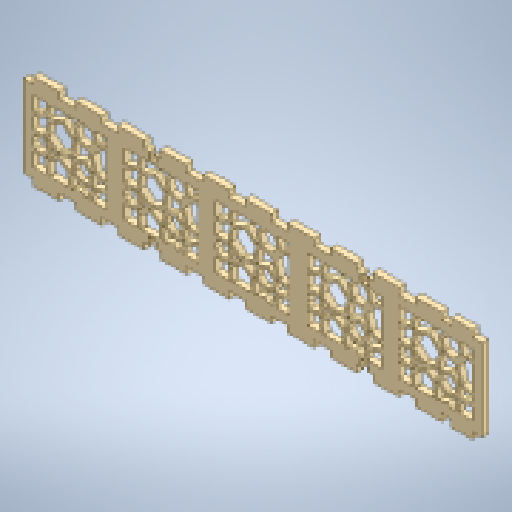
# Autodesk Inventor part: ширма
Saved by Autodesk Inventor 2023.1 (Build 271208000, 208)
## iProperties
Created: 2026-02-21
Part Number: ширма
Material: Типовые
Document SubType Name: Modeling
Designer: DELL
Density: 1 g/cm^3
Appearance: Пшеничный
Author: DELL
Autodesk Inventor part; units mm, degrees
ref_plane "YZ Plane" through (0, 0, 0) normal (1, 0, 0) x (0, 1, 0)
ref_plane "XZ Plane" through (0, 0, 0) normal (0, 1, 0) x (-1, 0, 0)
ref_plane "XY Plane" through (0, 0, 0) normal (0, 0, 1) x (1, 0, 0)
sketch "Эскиз1" plane through (0, 0, 0) normal (0, 0, 1) x (1, 0, 0)
  line L0 (-140.4, 25) -> (140.4, 25)
  line L1 (140.4, 25) -> (140.4, -25)
  line L2 (140.4, -25) -> (-140.4, -25)
  line L3 (-140.4, -25) -> (-140.4, 25)
  line L4 (-140.4, 25) -> (140.4, -25) construction
  line L5 (140.4, 25) -> (-140.4, -25) construction
  line L6 (-140.4, 0) -> (140.4, 0) construction
  line L7 (-140.4, 25) -> (-85.2, 25)
  line L8 (-85.2, 25) -> (-85.2, -25) construction
  line L9 (-85.2, -25) -> (-140.4, -25)
  line L10 (-140.4, -25) -> (-140.4, 25)
  line L11 (-89.2, -19) -> (-89.2, 19)
  line L12 (-89.2, 19) -> (-134.4, 19)
  line L13 (-134.4, 19) -> (-134.4, -19)
  line L14 (-134.4, -19) -> (-89.2, -19)
  line L15 (-125.4633, 11.2727) -> (-134.4, 8.1691)
  line L16 (-136.6237, 7.3969) -> (-145.5604, 15.1242) construction
  line L17 (-145.5604, 15.1242) -> (-143.3367, 26.7273) construction
  line L18 (-143.3367, 26.7273) -> (-132.1763, 30.6031) construction
  line L19 (-132.1763, 30.6031) -> (-123.2396, 22.8758) construction
  line L20 (-123.2396, 22.8758) -> (-123.9824, 19) construction
  line L21 (-127.2102, 12.7832) -> (-134.4, 10.2863)
  line L22 (-136.189, 9.665) -> (-143.3788, 15.8818) construction
  line L23 (-143.3788, 15.8818) -> (-141.5898, 25.2168) construction
  line L24 (-141.5898, 25.2168) -> (-132.611, 28.335) construction
  line L25 (-132.611, 28.335) -> (-125.4212, 22.1182) construction
  line L26 (-125.4212, 22.1182) -> (-126.0188, 19) construction
  line L27 (-107.9318, 7.9129) -> (-109.8716, -2.2089)
  line L28 (-109.8716, -2.2089) -> (-119.6072, -5.5899)
  line L29 (-119.6072, -5.5899) -> (-127.4031, 1.1509)
  line L30 (-127.4031, 1.1509) -> (-125.4633, 11.2727)
  line L31 (-125.4633, 11.2727) -> (-115.7276, 14.6537)
  line L32 (-115.7276, 14.6537) -> (-107.9318, 7.9129)
  line L33 (-116.1623, 12.3855) -> (-110.1134, 7.1552)
  line L34 (-110.1134, 7.1552) -> (-111.6185, -0.6984)
  line L35 (-111.6185, -0.6984) -> (-119.1726, -3.3218)
  line L36 (-119.1726, -3.3218) -> (-125.2215, 1.9085)
  line L37 (-125.2215, 1.9085) -> (-123.7163, 9.7622)
  line L38 (-123.7163, 9.7622) -> (-116.1623, 12.3855)
  line L39 (-102.8211, 0.2395) -> (-97.1755, -4.6421)
  line L40 (-97.1755, -4.6421) -> (-98.5803, -11.9722)
  line L41 (-98.5803, -11.9722) -> (-105.6307, -14.4207)
  line L42 (-105.6307, -14.4207) -> (-111.2764, -9.539)
  line L43 (-111.2764, -9.539) -> (-109.8716, -2.2089)
  line L44 (-109.8716, -2.2089) -> (-102.8211, 0.2395)
  line L45 (-103.2558, -2.0286) -> (-99.3571, -5.3997)
  line L46 (-99.3571, -5.3997) -> (-100.3272, -10.4617)
  line L47 (-100.3272, -10.4617) -> (-105.196, -12.1525)
  line L48 (-105.196, -12.1525) -> (-109.0948, -8.7814)
  line L49 (-109.0948, -8.7814) -> (-108.1247, -3.7194)
  line L50 (-108.1247, -3.7194) -> (-103.2558, -2.0286)
  line L51 (-98.5803, -11.9722) -> (-89.2, -8.7146)
  line L52 (-89.9827, -8.9864) -> (-83.0982, -14.9393) construction
  line L53 (-83.0982, -14.9393) -> (-84.8112, -23.8778) construction
  line L54 (-84.8112, -23.8778) -> (-93.4088, -26.8636) construction
  line L55 (-93.4088, -26.8636) -> (-102.5031, -19) construction
  line L56 (-100.2933, -20.9108) -> (-98.5803, -11.9722)
  line L57 (-90.4174, -11.2546) -> (-89.2, -12.3072)
  line L58 (-85.2798, -15.6969) -> (-86.5582, -22.3673) construction
  line L59 (-86.5582, -22.3673) -> (-92.9741, -24.5955) construction
  line L60 (-92.9741, -24.5955) -> (-99.4453, -19) construction
  line L61 (-98.1117, -20.1531) -> (-96.8333, -13.4827)
  line L62 (-96.8333, -13.4827) -> (-90.4174, -11.2546)
  line L63 (-110.531, -18.7283) -> (-110.9243, -19)
  line L64 (-118.1165, -23.9685) -> (-128.5977, -19) construction
  line L65 (-126.4473, -20.0194) -> (-127.1927, -10.8301)
  line L66 (-127.1927, -10.8301) -> (-119.6072, -5.5899)
  line L67 (-119.6072, -5.5899) -> (-111.2764, -9.539)
  line L68 (-111.2764, -9.539) -> (-110.531, -18.7283)
  line L69 (-118.3032, -21.6667) -> (-124.5472, -18.7068)
  line L70 (-124.5472, -18.7068) -> (-125.1059, -11.8193)
  line L71 (-125.1059, -11.8193) -> (-119.4205, -7.8918)
  line L72 (-119.4205, -7.8918) -> (-113.1765, -10.8517)
  line L73 (-113.1765, -10.8517) -> (-112.6178, -17.7391)
  line L74 (-112.6178, -17.7391) -> (-118.3032, -21.6667)
  line L75 (-104.7821, -16.8642) -> (-100.2933, -20.9108)
  line L76 (-100.2933, -20.9108) -> (-99.886, -19)
  line L77 (-101.5533, -26.8215) -> (-107.3022, -28.6856) construction
  line L78 (-107.3022, -28.6856) -> (-111.791, -24.6391) construction
  line L79 (-111.791, -24.6391) -> (-110.5889, -19)
  line L80 (-110.531, -18.7283) -> (-104.7821, -16.8642)
  line L81 (-105.2636, -19.1228) -> (-102.4901, -21.6231)
  line L82 (-102.4901, -21.6231) -> (-101.9309, -19)
  line L83 (-103.2686, -25.2752) -> (-106.8207, -26.427) construction
  line L84 (-106.8207, -26.427) -> (-109.5942, -23.9267) construction
  line L85 (-109.5942, -23.9267) -> (-108.544, -19) construction
  line L86 (-108.8157, -20.2746) -> (-105.2636, -19.1228)
  line L87 (-107.9318, 7.9129) -> (-110.126, 15.5167)
  line L88 (-110.126, 15.5167) -> (-106.7735, 19)
  line L89 (-104.6379, 21.2189) -> (-96.9557, 19.3171) construction
  line L90 (-96.9557, 19.3171) -> (-96.8642, 19)
  line L91 (-94.7615, 11.7133) -> (-100.2496, 6.0111)
  line L92 (-100.2496, 6.0111) -> (-107.9318, 7.9129)
  line L93 (-106.3303, 9.5768) -> (-107.8842, 14.9618)
  line L94 (-107.8842, 14.9618) -> (-103.9976, 19)
  line L95 (-103.9976, 19) -> (-98.5571, 17.6532)
  line L96 (-98.5571, 17.6532) -> (-97.0032, 12.2682)
  line L97 (-97.0032, 12.2682) -> (-100.8898, 8.23)
  line L98 (-100.8898, 8.23) -> (-106.3303, 9.5768)
  line L99 (-97.1755, -4.6421) -> (-100.2496, 6.0111)
  line L100 (-100.2496, 6.0111) -> (-92.5607, 14)
  line L101 (-92.5607, 14) -> (-89.2, 13.1681)
  line L102 (-81.7977, 11.3356) -> (-78.7236, 0.6824) construction
  line L103 (-78.7236, 0.6824) -> (-86.4125, -7.3065) construction
  line L104 (-86.4125, -7.3065) -> (-89.2, -6.6164) construction
  line L105 (-98.0078, 5.4562) -> (-91.9204, 11.7811)
  line L106 (-91.9204, 11.7811) -> (-89.2, 11.1077)
  line L107 (-83.3991, 9.6717) -> (-80.9653, 1.2373) construction
  line L108 (-80.9653, 1.2373) -> (-87.0528, -5.0876) construction
  line L109 (-87.0528, -5.0876) -> (-89.2, -4.556) construction
  line L110 (-95.574, -2.9782) -> (-98.0078, 5.4562)
  line L111 (-123.8393, -4.7789) -> (-127.1927, -10.8301)
  line L112 (-127.1927, -10.8301) -> (-134.1099, -10.9515)
  line L113 (-134.1099, -10.9515) -> (-134.4, -10.4689)
  line L114 (-137.6737, -5.0218) -> (-134.4, 0.8856) construction
  line L115 (-134.3203, 1.0294) -> (-127.4031, 1.1509)
  line L116 (-127.4031, 1.1509) -> (-123.8393, -4.7789)
  line L117 (-128.5225, -0.8691) -> (-126.1483, -4.8194)
  line L118 (-126.1483, -4.8194) -> (-128.3823, -8.8507)
  line L119 (-128.3823, -8.8507) -> (-132.9905, -8.9316)
  line L120 (-132.9905, -8.9316) -> (-134.4, -6.5863)
  line L121 (-135.3647, -4.9812) -> (-134.4, -3.2405) construction
  line L122 (-133.1306, -0.95) -> (-128.5225, -0.8691)
  line L123 (-134.4, 10.2863) -> (-136.189, 9.665) construction
  line L124 (-134.4, 8.1691) -> (-136.6237, 7.3969) construction
  line L125 (-126.0188, 19) -> (-127.2102, 12.7832)
  line L126 (-123.9824, 19) -> (-125.4633, 11.2727)
  line L127 (-106.7735, 19) -> (-104.6379, 21.2189) construction
  line L128 (-96.8642, 19) -> (-94.7615, 11.7133)
  line L129 (-89.2, 13.1681) -> (-81.7977, 11.3356) construction
  line L130 (-89.2, 11.1077) -> (-83.3991, 9.6717) construction
  line L131 (-89.2, -4.556) -> (-95.574, -2.9782)
  line L132 (-89.2, -6.6164) -> (-97.1755, -4.6421)
  line L133 (-89.2, -8.7146) -> (-89.9827, -8.9864) construction
  line L134 (-89.2, -12.3072) -> (-85.2798, -15.6969) construction
  line L135 (-99.4453, -19) -> (-98.1117, -20.1531)
  line L136 (-102.5031, -19) -> (-100.2933, -20.9108)
  line L137 (-99.886, -19) -> (-101.5533, -26.8215) construction
  line L138 (-101.9309, -19) -> (-103.2686, -25.2752) construction
  line L139 (-108.544, -19) -> (-108.8157, -20.2746)
  line L140 (-110.5889, -19) -> (-110.531, -18.7283)
  line L141 (-110.9243, -19) -> (-118.1165, -23.9685) construction
  line L142 (-128.5977, -19) -> (-126.4473, -20.0194)
  line L143 (-134.4, -10.4689) -> (-137.6737, -5.0218) construction
  line L144 (-134.4, -6.5863) -> (-135.3647, -4.9812) construction
  line L145 (-134.4, -3.2405) -> (-133.1306, -0.95)
  line L146 (-134.4, 0.8856) -> (-134.3203, 1.0294)
  line L147 (-72.5977, -19) -> (-70.4473, -20.0194)
  line L148 (-62.3032, -21.6667) -> (-68.5472, -18.7068)
  line L149 (-56.6178, -17.7391) -> (-62.3032, -21.6667)
  line L150 (-71.1927, -10.8301) -> (-63.6072, -5.5899)
  line L151 (-67.8393, -4.7789) -> (-71.1927, -10.8301)
  line L152 (-71.1927, -10.8301) -> (-78.1099, -10.9515)
  line L153 (-70.1483, -4.8194) -> (-72.3823, -8.8507)
  line L154 (-72.3823, -8.8507) -> (-76.9905, -8.9316)
  line L155 (-76.9905, -8.9316) -> (-78.4, -6.5863)
  line L156 (-78.1099, -10.9515) -> (-78.4, -10.4689)
  line L157 (-78.4, -3.2405) -> (-77.1306, -0.95)
  line L158 (-55.2764, -9.539) -> (-54.531, -18.7283)
  line L159 (-54.5889, -19) -> (-54.531, -18.7283)
  line L160 (-54.531, -18.7283) -> (-48.7821, -16.8642)
  line L161 (-52.544, -19) -> (-52.8157, -20.2746)
  line L162 (-52.8157, -20.2746) -> (-49.2636, -19.1228)
  line L163 (-78.3203, 1.0294) -> (-71.4031, 1.1509)
  line L164 (-78.4, 0.8856) -> (-78.3203, 1.0294)
  line L165 (-77.1306, -0.95) -> (-72.5225, -0.8691)
  line L166 (-72.5225, -0.8691) -> (-70.1483, -4.8194)
  line L167 (-63.1726, -3.3218) -> (-69.2215, 1.9085)
  line L168 (-63.6072, -5.5899) -> (-71.4031, 1.1509)
  line L169 (-71.4031, 1.1509) -> (-67.8393, -4.7789)
  line L170 (-53.8716, -2.2089) -> (-63.6072, -5.5899)
  line L171 (-55.6185, -0.6984) -> (-63.1726, -3.3218)
  line L172 (-49.6307, -14.4207) -> (-55.2764, -9.539)
  line L173 (-55.2764, -9.539) -> (-53.8716, -2.2089)
  line L174 (-63.6072, -5.5899) -> (-55.2764, -9.539)
  line L175 (-53.0948, -8.7814) -> (-52.1247, -3.7194)
  line L176 (-49.196, -12.1525) -> (-53.0948, -8.7814)
  line L177 (-63.4205, -7.8918) -> (-57.1765, -10.8517)
  line L178 (-69.2215, 1.9085) -> (-67.7163, 9.7622)
  line L179 (-71.4031, 1.1509) -> (-69.4633, 11.2727)
  line L180 (-67.7163, 9.7622) -> (-60.1623, 12.3855)
  line L181 (-69.4633, 11.2727) -> (-59.7276, 14.6537)
  line L182 (-69.4633, 11.2727) -> (-78.4, 8.1691)
  line L183 (-71.2102, 12.7832) -> (-78.4, 10.2863)
  line L184 (-42.5803, -11.9722) -> (-49.6307, -14.4207)
  line L185 (-44.3272, -10.4617) -> (-49.196, -12.1525)
  line L186 (-42.1117, -20.1531) -> (-40.8333, -13.4827)
  line L187 (-44.2933, -20.9108) -> (-42.5803, -11.9722)
  line L188 (-46.5031, -19) -> (-44.2933, -20.9108)
  line L189 (-44.2933, -20.9108) -> (-43.886, -19)
  line L190 (-46.4901, -21.6231) -> (-45.9309, -19)
  line L191 (-49.2636, -19.1228) -> (-46.4901, -21.6231)
  line L192 (-48.7821, -16.8642) -> (-44.2933, -20.9108)
  line L193 (-43.4453, -19) -> (-42.1117, -20.1531)
  line L194 (-78.4, 19) -> (-78.4, -19)
  line L195 (-41.1755, -4.6421) -> (-42.5803, -11.9722)
  line L196 (-43.3571, -5.3997) -> (-44.3272, -10.4617)
  line L197 (-42.5803, -11.9722) -> (-33.2, -8.7146)
  line L198 (-34.4174, -11.2546) -> (-33.2, -12.3072)
  line L199 (-40.8333, -13.4827) -> (-34.4174, -11.2546)
  line L200 (-51.9318, 7.9129) -> (-53.8716, -2.2089)
  line L201 (-59.7276, 14.6537) -> (-51.9318, 7.9129)
  line L202 (-60.1623, 12.3855) -> (-54.1134, 7.1552)
  line L203 (-54.1134, 7.1552) -> (-55.6185, -0.6984)
  line L204 (-50.3303, 9.5768) -> (-51.8842, 14.9618)
  line L205 (-51.9318, 7.9129) -> (-54.126, 15.5167)
  line L206 (-44.8898, 8.23) -> (-50.3303, 9.5768)
  line L207 (-44.2496, 6.0111) -> (-51.9318, 7.9129)
  line L208 (-41.0032, 12.2682) -> (-44.8898, 8.23)
  line L209 (-44.2496, 6.0111) -> (-36.5607, 14)
  line L210 (-53.8716, -2.2089) -> (-46.8211, 0.2395)
  line L211 (-52.1247, -3.7194) -> (-47.2558, -2.0286)
  line L212 (-47.2558, -2.0286) -> (-43.3571, -5.3997)
  line L213 (-46.8211, 0.2395) -> (-41.1755, -4.6421)
  line L214 (-42.0078, 5.4562) -> (-35.9204, 11.7811)
  line L215 (-40.8642, 19) -> (-38.7615, 11.7133)
  line L216 (-42.5571, 17.6532) -> (-41.0032, 12.2682)
  line L217 (-47.9976, 19) -> (-42.5571, 17.6532)
  line L218 (-40.9557, 19.3171) -> (-40.8642, 19)
  line L219 (-51.8842, 14.9618) -> (-47.9976, 19)
  line L220 (-54.126, 15.5167) -> (-50.7735, 19)
  line L221 (-38.7615, 11.7133) -> (-44.2496, 6.0111)
  line L222 (-33.2, -6.6164) -> (-41.1755, -4.6421)
  line L223 (-33.2, -4.556) -> (-39.574, -2.9782)
  line L224 (-41.1755, -4.6421) -> (-44.2496, 6.0111)
  line L225 (-39.574, -2.9782) -> (-42.0078, 5.4562)
  line L226 (-35.9204, 11.7811) -> (-33.2, 11.1077)
  line L227 (-36.5607, 14) -> (-33.2, 13.1681)
  line L228 (-68.5472, -18.7068) -> (-69.1059, -11.8193)
  line L229 (-54.531, -18.7283) -> (-54.9243, -19)
  line L230 (-69.1059, -11.8193) -> (-63.4205, -7.8918)
  line L231 (-57.1765, -10.8517) -> (-56.6178, -17.7391)
  line L232 (-78.4, -19) -> (-33.2, -19)
  line L233 (-33.2, -19) -> (-33.2, 19)
  line L234 (-33.2, 19) -> (-78.4, 19)
  line L235 (-70.4473, -20.0194) -> (-71.1927, -10.8301)
  line L236 (-67.9824, 19) -> (-69.4633, 11.2727)
  line L237 (-70.0188, 19) -> (-71.2102, 12.7832)
  line L238 (-16.5977, -19) -> (-14.4473, -20.0194)
  line L239 (-6.3032, -21.6667) -> (-12.5472, -18.7068)
  line L240 (-0.6178, -17.7391) -> (-6.3032, -21.6667)
  line L241 (-15.1927, -10.8301) -> (-7.6072, -5.5899)
  line L242 (-11.8393, -4.7789) -> (-15.1927, -10.8301)
  line L243 (-15.1927, -10.8301) -> (-22.1099, -10.9515)
  line L244 (-14.1483, -4.8194) -> (-16.3823, -8.8507)
  line L245 (-16.3823, -8.8507) -> (-20.9905, -8.9316)
  line L246 (-20.9905, -8.9316) -> (-22.4, -6.5863)
  line L247 (-22.1099, -10.9515) -> (-22.4, -10.4689)
  line L248 (-22.4, -3.2405) -> (-21.1306, -0.95)
  line L249 (0.7236, -9.539) -> (1.469, -18.7283)
  line L250 (1.4111, -19) -> (1.469, -18.7283)
  line L251 (1.469, -18.7283) -> (7.2179, -16.8642)
  line L252 (3.456, -19) -> (3.1843, -20.2746)
  line L253 (3.1843, -20.2746) -> (6.7364, -19.1228)
  line L254 (-22.3203, 1.0294) -> (-15.4031, 1.1509)
  line L255 (-22.4, 0.8856) -> (-22.3203, 1.0294)
  line L256 (-21.1306, -0.95) -> (-16.5225, -0.8691)
  line L257 (-16.5225, -0.8691) -> (-14.1483, -4.8194)
  line L258 (-7.1726, -3.3218) -> (-13.2215, 1.9085)
  line L259 (-7.6072, -5.5899) -> (-15.4031, 1.1509)
  line L260 (-15.4031, 1.1509) -> (-11.8393, -4.7789)
  line L261 (2.1284, -2.2089) -> (-7.6072, -5.5899)
  line L262 (0.3815, -0.6984) -> (-7.1726, -3.3218)
  line L263 (6.3693, -14.4207) -> (0.7236, -9.539)
  line L264 (0.7236, -9.539) -> (2.1284, -2.2089)
  line L265 (-7.6072, -5.5899) -> (0.7236, -9.539)
  line L266 (2.9052, -8.7814) -> (3.8753, -3.7194)
  line L267 (6.804, -12.1525) -> (2.9052, -8.7814)
  line L268 (-7.4205, -7.8918) -> (-1.1765, -10.8517)
  line L269 (-13.2215, 1.9085) -> (-11.7163, 9.7622)
  line L270 (-15.4031, 1.1509) -> (-13.4633, 11.2727)
  line L271 (-11.7163, 9.7622) -> (-4.1623, 12.3855)
  line L272 (-13.4633, 11.2727) -> (-3.7276, 14.6537)
  line L273 (-13.4633, 11.2727) -> (-22.4, 8.1691)
  line L274 (-15.2102, 12.7832) -> (-22.4, 10.2863)
  line L275 (13.4197, -11.9722) -> (6.3693, -14.4207)
  line L276 (11.6728, -10.4617) -> (6.804, -12.1525)
  line L277 (13.8883, -20.1531) -> (15.1667, -13.4827)
  line L278 (11.7067, -20.9108) -> (13.4197, -11.9722)
  line L279 (9.4969, -19) -> (11.7067, -20.9108)
  line L280 (11.7067, -20.9108) -> (12.114, -19)
  line L281 (9.5099, -21.6231) -> (10.0691, -19)
  line L282 (6.7364, -19.1228) -> (9.5099, -21.6231)
  line L283 (7.2179, -16.8642) -> (11.7067, -20.9108)
  line L284 (12.5547, -19) -> (13.8883, -20.1531)
  line L285 (-22.4, 19) -> (-22.4, -19)
  line L286 (14.8245, -4.6421) -> (13.4197, -11.9722)
  line L287 (12.6429, -5.3997) -> (11.6728, -10.4617)
  line L288 (13.4197, -11.9722) -> (22.8, -8.7146)
  line L289 (21.5826, -11.2546) -> (22.8, -12.3072)
  line L290 (15.1667, -13.4827) -> (21.5826, -11.2546)
  line L291 (4.0682, 7.9129) -> (2.1284, -2.2089)
  line L292 (-3.7276, 14.6537) -> (4.0682, 7.9129)
  line L293 (-4.1623, 12.3855) -> (1.8866, 7.1552)
  line L294 (1.8866, 7.1552) -> (0.3815, -0.6984)
  line L295 (5.6697, 9.5768) -> (4.1158, 14.9618)
  line L296 (4.0682, 7.9129) -> (1.874, 15.5167)
  line L297 (11.1102, 8.23) -> (5.6697, 9.5768)
  line L298 (11.7504, 6.0111) -> (4.0682, 7.9129)
  line L299 (14.9968, 12.2682) -> (11.1102, 8.23)
  line L300 (11.7504, 6.0111) -> (19.4393, 14)
  line L301 (2.1284, -2.2089) -> (9.1789, 0.2395)
  line L302 (3.8753, -3.7194) -> (8.7442, -2.0286)
  line L303 (8.7442, -2.0286) -> (12.6429, -5.3997)
  line L304 (9.1789, 0.2395) -> (14.8245, -4.6421)
  line L305 (13.9922, 5.4562) -> (20.0796, 11.7811)
  line L306 (15.1358, 19) -> (17.2385, 11.7133)
  line L307 (13.4429, 17.6532) -> (14.9968, 12.2682)
  line L308 (8.0024, 19) -> (13.4429, 17.6532)
  line L309 (15.0443, 19.3171) -> (15.1358, 19)
  line L310 (4.1158, 14.9618) -> (8.0024, 19)
  line L311 (1.874, 15.5167) -> (5.2265, 19)
  line L312 (17.2385, 11.7133) -> (11.7504, 6.0111)
  line L313 (22.8, -6.6164) -> (14.8245, -4.6421)
  line L314 (22.8, -4.556) -> (16.426, -2.9782)
  line L315 (14.8245, -4.6421) -> (11.7504, 6.0111)
  line L316 (16.426, -2.9782) -> (13.9922, 5.4562)
  line L317 (20.0796, 11.7811) -> (22.8, 11.1077)
  line L318 (19.4393, 14) -> (22.8, 13.1681)
  line L319 (-12.5472, -18.7068) -> (-13.1059, -11.8193)
  line L320 (1.469, -18.7283) -> (1.0757, -19)
  line L321 (-13.1059, -11.8193) -> (-7.4205, -7.8918)
  line L322 (-1.1765, -10.8517) -> (-0.6178, -17.7391)
  line L323 (-22.4, -19) -> (22.8, -19)
  line L324 (22.8, -19) -> (22.8, 19)
  line L325 (22.8, 19) -> (-22.4, 19)
  line L326 (-14.4473, -20.0194) -> (-15.1927, -10.8301)
  line L327 (-11.9824, 19) -> (-13.4633, 11.2727)
  line L328 (-14.0188, 19) -> (-15.2102, 12.7832)
  line L329 (39.4023, -19) -> (41.5527, -20.0194)
  line L330 (49.6968, -21.6667) -> (43.4528, -18.7068)
  line L331 (55.3822, -17.7391) -> (49.6968, -21.6667)
  line L332 (40.8073, -10.8301) -> (48.3928, -5.5899)
  line L333 (44.1607, -4.7789) -> (40.8073, -10.8301)
  line L334 (40.8073, -10.8301) -> (33.8901, -10.9515)
  line L335 (41.8517, -4.8194) -> (39.6177, -8.8507)
  line L336 (39.6177, -8.8507) -> (35.0095, -8.9316)
  line L337 (35.0095, -8.9316) -> (33.6, -6.5863)
  line L338 (33.8901, -10.9515) -> (33.6, -10.4689)
  line L339 (33.6, -3.2405) -> (34.8694, -0.95)
  line L340 (56.7236, -9.539) -> (57.469, -18.7283)
  line L341 (57.4111, -19) -> (57.469, -18.7283)
  line L342 (57.469, -18.7283) -> (63.2179, -16.8642)
  line L343 (59.456, -19) -> (59.1843, -20.2746)
  line L344 (59.1843, -20.2746) -> (62.7364, -19.1228)
  line L345 (33.6797, 1.0294) -> (40.5969, 1.1509)
  line L346 (33.6, 0.8856) -> (33.6797, 1.0294)
  line L347 (34.8694, -0.95) -> (39.4775, -0.8691)
  line L348 (39.4775, -0.8691) -> (41.8517, -4.8194)
  line L349 (48.8274, -3.3218) -> (42.7785, 1.9085)
  line L350 (48.3928, -5.5899) -> (40.5969, 1.1509)
  line L351 (40.5969, 1.1509) -> (44.1607, -4.7789)
  line L352 (58.1284, -2.2089) -> (48.3928, -5.5899)
  line L353 (56.3815, -0.6984) -> (48.8274, -3.3218)
  line L354 (62.3693, -14.4207) -> (56.7236, -9.539)
  line L355 (56.7236, -9.539) -> (58.1284, -2.2089)
  line L356 (48.3928, -5.5899) -> (56.7236, -9.539)
  line L357 (58.9052, -8.7814) -> (59.8753, -3.7194)
  line L358 (62.804, -12.1525) -> (58.9052, -8.7814)
  line L359 (48.5795, -7.8918) -> (54.8235, -10.8517)
  line L360 (42.7785, 1.9085) -> (44.2837, 9.7622)
  line L361 (40.5969, 1.1509) -> (42.5367, 11.2727)
  line L362 (44.2837, 9.7622) -> (51.8377, 12.3855)
  line L363 (42.5367, 11.2727) -> (52.2724, 14.6537)
  line L364 (42.5367, 11.2727) -> (33.6, 8.1691)
  line L365 (40.7898, 12.7832) -> (33.6, 10.2863)
  line L366 (69.4197, -11.9722) -> (62.3693, -14.4207)
  line L367 (67.6728, -10.4617) -> (62.804, -12.1525)
  line L368 (69.8883, -20.1531) -> (71.1667, -13.4827)
  line L369 (67.7067, -20.9108) -> (69.4197, -11.9722)
  line L370 (65.4969, -19) -> (67.7067, -20.9108)
  line L371 (67.7067, -20.9108) -> (68.114, -19)
  line L372 (65.5099, -21.6231) -> (66.0691, -19)
  line L373 (62.7364, -19.1228) -> (65.5099, -21.6231)
  line L374 (63.2179, -16.8642) -> (67.7067, -20.9108)
  line L375 (68.5547, -19) -> (69.8883, -20.1531)
  line L376 (33.6, 19) -> (33.6, -19)
  line L377 (70.8245, -4.6421) -> (69.4197, -11.9722)
  line L378 (68.6429, -5.3997) -> (67.6728, -10.4617)
  line L379 (69.4197, -11.9722) -> (78.8, -8.7146)
  line L380 (77.5826, -11.2546) -> (78.8, -12.3072)
  line L381 (71.1667, -13.4827) -> (77.5826, -11.2546)
  line L382 (60.0682, 7.9129) -> (58.1284, -2.2089)
  line L383 (52.2724, 14.6537) -> (60.0682, 7.9129)
  line L384 (51.8377, 12.3855) -> (57.8866, 7.1552)
  line L385 (57.8866, 7.1552) -> (56.3815, -0.6984)
  line L386 (61.6697, 9.5768) -> (60.1158, 14.9618)
  line L387 (60.0682, 7.9129) -> (57.874, 15.5167)
  line L388 (67.1102, 8.23) -> (61.6697, 9.5768)
  line L389 (67.7504, 6.0111) -> (60.0682, 7.9129)
  line L390 (70.9968, 12.2682) -> (67.1102, 8.23)
  line L391 (67.7504, 6.0111) -> (75.4393, 14)
  line L392 (58.1284, -2.2089) -> (65.1789, 0.2395)
  line L393 (59.8753, -3.7194) -> (64.7442, -2.0286)
  line L394 (64.7442, -2.0286) -> (68.6429, -5.3997)
  line L395 (65.1789, 0.2395) -> (70.8245, -4.6421)
  line L396 (69.9922, 5.4562) -> (76.0796, 11.7811)
  line L397 (71.1358, 19) -> (73.2385, 11.7133)
  line L398 (69.4429, 17.6532) -> (70.9968, 12.2682)
  line L399 (64.0024, 19) -> (69.4429, 17.6532)
  line L400 (71.0443, 19.3171) -> (71.1358, 19)
  line L401 (60.1158, 14.9618) -> (64.0024, 19)
  line L402 (57.874, 15.5167) -> (61.2265, 19)
  line L403 (73.2385, 11.7133) -> (67.7504, 6.0111)
  line L404 (78.8, -6.6164) -> (70.8245, -4.6421)
  line L405 (78.8, -4.556) -> (72.426, -2.9782)
  line L406 (70.8245, -4.6421) -> (67.7504, 6.0111)
  line L407 (72.426, -2.9782) -> (69.9922, 5.4562)
  line L408 (76.0796, 11.7811) -> (78.8, 11.1077)
  line L409 (75.4393, 14) -> (78.8, 13.1681)
  line L410 (43.4528, -18.7068) -> (42.8941, -11.8193)
  line L411 (57.469, -18.7283) -> (57.0757, -19)
  line L412 (42.8941, -11.8193) -> (48.5795, -7.8918)
  line L413 (54.8235, -10.8517) -> (55.3822, -17.7391)
  line L414 (33.6, -19) -> (78.8, -19)
  line L415 (78.8, -19) -> (78.8, 19)
  line L416 (78.8, 19) -> (33.6, 19)
  line L417 (41.5527, -20.0194) -> (40.8073, -10.8301)
  line L418 (44.0176, 19) -> (42.5367, 11.2727)
  line L419 (41.9812, 19) -> (40.7898, 12.7832)
  line L420 (95.4023, -19) -> (97.5527, -20.0194)
  line L421 (105.6968, -21.6667) -> (99.4528, -18.7068)
  line L422 (111.3822, -17.7391) -> (105.6968, -21.6667)
  line L423 (96.8073, -10.8301) -> (104.3928, -5.5899)
  line L424 (100.1607, -4.7789) -> (96.8073, -10.8301)
  line L425 (96.8073, -10.8301) -> (89.8901, -10.9515)
  line L426 (97.8517, -4.8194) -> (95.6177, -8.8507)
  line L427 (95.6177, -8.8507) -> (91.0095, -8.9316)
  line L428 (91.0095, -8.9316) -> (89.6, -6.5863)
  line L429 (89.8901, -10.9515) -> (89.6, -10.4689)
  line L430 (89.6, -3.2405) -> (90.8694, -0.95)
  line L431 (112.7236, -9.539) -> (113.469, -18.7283)
  line L432 (113.4111, -19) -> (113.469, -18.7283)
  line L433 (113.469, -18.7283) -> (119.2179, -16.8642)
  line L434 (115.456, -19) -> (115.1843, -20.2746)
  line L435 (115.1843, -20.2746) -> (118.7364, -19.1228)
  line L436 (89.6797, 1.0294) -> (96.5969, 1.1509)
  line L437 (89.6, 0.8856) -> (89.6797, 1.0294)
  line L438 (90.8694, -0.95) -> (95.4775, -0.8691)
  line L439 (95.4775, -0.8691) -> (97.8517, -4.8194)
  line L440 (104.8274, -3.3218) -> (98.7785, 1.9085)
  line L441 (104.3928, -5.5899) -> (96.5969, 1.1509)
  line L442 (96.5969, 1.1509) -> (100.1607, -4.7789)
  line L443 (114.1284, -2.2089) -> (104.3928, -5.5899)
  line L444 (112.3815, -0.6984) -> (104.8274, -3.3218)
  line L445 (118.3693, -14.4207) -> (112.7236, -9.539)
  line L446 (112.7236, -9.539) -> (114.1284, -2.2089)
  line L447 (104.3928, -5.5899) -> (112.7236, -9.539)
  line L448 (114.9052, -8.7814) -> (115.8753, -3.7194)
  line L449 (118.804, -12.1525) -> (114.9052, -8.7814)
  line L450 (104.5795, -7.8918) -> (110.8235, -10.8517)
  line L451 (98.7785, 1.9085) -> (100.2837, 9.7622)
  line L452 (96.5969, 1.1509) -> (98.5367, 11.2727)
  line L453 (100.2837, 9.7622) -> (107.8377, 12.3855)
  line L454 (98.5367, 11.2727) -> (108.2724, 14.6537)
  line L455 (98.5367, 11.2727) -> (89.6, 8.1691)
  line L456 (96.7898, 12.7832) -> (89.6, 10.2863)
  line L457 (125.4197, -11.9722) -> (118.3693, -14.4207)
  line L458 (123.6728, -10.4617) -> (118.804, -12.1525)
  line L459 (125.8883, -20.1531) -> (127.1667, -13.4827)
  line L460 (123.7067, -20.9108) -> (125.4197, -11.9722)
  line L461 (121.4969, -19) -> (123.7067, -20.9108)
  line L462 (123.7067, -20.9108) -> (124.114, -19)
  line L463 (121.5099, -21.6231) -> (122.0691, -19)
  line L464 (118.7364, -19.1228) -> (121.5099, -21.6231)
  line L465 (119.2179, -16.8642) -> (123.7067, -20.9108)
  line L466 (124.5547, -19) -> (125.8883, -20.1531)
  line L467 (89.6, 19) -> (89.6, -19)
  line L468 (126.8245, -4.6421) -> (125.4197, -11.9722)
  line L469 (124.6429, -5.3997) -> (123.6728, -10.4617)
  line L470 (125.4197, -11.9722) -> (134.8, -8.7146)
  line L471 (133.5826, -11.2546) -> (134.8, -12.3072)
  line L472 (127.1667, -13.4827) -> (133.5826, -11.2546)
  line L473 (116.0682, 7.9129) -> (114.1284, -2.2089)
  line L474 (108.2724, 14.6537) -> (116.0682, 7.9129)
  line L475 (107.8377, 12.3855) -> (113.8866, 7.1552)
  line L476 (113.8866, 7.1552) -> (112.3815, -0.6984)
  line L477 (117.6697, 9.5768) -> (116.1158, 14.9618)
  line L478 (116.0682, 7.9129) -> (113.874, 15.5167)
  line L479 (123.1102, 8.23) -> (117.6697, 9.5768)
  line L480 (123.7504, 6.0111) -> (116.0682, 7.9129)
  line L481 (126.9968, 12.2682) -> (123.1102, 8.23)
  line L482 (123.7504, 6.0111) -> (131.4393, 14)
  line L483 (114.1284, -2.2089) -> (121.1789, 0.2395)
  line L484 (115.8753, -3.7194) -> (120.7442, -2.0286)
  line L485 (120.7442, -2.0286) -> (124.6429, -5.3997)
  line L486 (121.1789, 0.2395) -> (126.8245, -4.6421)
  line L487 (125.9922, 5.4562) -> (132.0796, 11.7811)
  line L488 (127.1358, 19) -> (129.2385, 11.7133)
  line L489 (125.4429, 17.6532) -> (126.9968, 12.2682)
  line L490 (120.0024, 19) -> (125.4429, 17.6532)
  line L491 (127.0443, 19.3171) -> (127.1358, 19)
  line L492 (116.1158, 14.9618) -> (120.0024, 19)
  line L493 (113.874, 15.5167) -> (117.2265, 19)
  line L494 (129.2385, 11.7133) -> (123.7504, 6.0111)
  line L495 (134.8, -6.6164) -> (126.8245, -4.6421)
  line L496 (134.8, -4.556) -> (128.426, -2.9782)
  line L497 (126.8245, -4.6421) -> (123.7504, 6.0111)
  line L498 (128.426, -2.9782) -> (125.9922, 5.4562)
  line L499 (132.0796, 11.7811) -> (134.8, 11.1077)
  line L500 (131.4393, 14) -> (134.8, 13.1681)
  line L501 (99.4528, -18.7068) -> (98.8941, -11.8193)
  line L502 (113.469, -18.7283) -> (113.0757, -19)
  line L503 (98.8941, -11.8193) -> (104.5795, -7.8918)
  line L504 (110.8235, -10.8517) -> (111.3822, -17.7391)
  line L505 (89.6, -19) -> (134.8, -19)
  line L506 (134.8, -19) -> (134.8, 19)
  line L507 (134.8, 19) -> (89.6, 19)
  line L508 (97.5527, -20.0194) -> (96.8073, -10.8301)
  line L509 (100.0176, 19) -> (98.5367, 11.2727)
  line L510 (97.9812, 19) -> (96.7898, 12.7832)
  point P0 (0, 0)
  point P1 (-117.6674, 4.5319)
  point P2 (-117.6674, 4.5319)
  point P3 (-104.2259, -7.0906)
  point P4 (-104.2259, -7.0906)
  point P5 (-91.6958, -17.925)
  point P6 (-91.6958, -17.925)
  point P7 (-60.2815, -8.4793)
  point P8 (-93.6254, -12.3686)
  point P9 (-118.8618, -14.7792)
  point P10 (-118.8618, -14.7792)
  point P11 (-106.0422, -22.7749)
  point P12 (-106.0422, -22.7749)
  point P13 (-102.4437, 13.615)
  point P14 (-102.4437, 13.615)
  point P15 (-89.4866, 3.3468)
  point P16 (-89.4866, 3.3468)
  point P17 (-130.7565, -4.9003)
  point P18 (-130.7565, -4.9003)
  point P19 (-62.1165, -23.9685)
  point P20 (-62.8618, -14.7792)
  point P21 (-62.8618, -14.7792)
  point P22 (-74.7565, -4.9003)
  point P23 (-53.5942, -23.9267)
  point P24 (-61.6674, 4.5319)
  point P25 (-61.6674, 4.5319)
  point P26 (-74.7565, -4.9003)
  point P27 (-48.2259, -7.0906)
  point P28 (-48.2259, -7.0906)
  point P29 (-50.0422, -22.7749)
  point P30 (-50.0422, -22.7749)
  point P31 (-35.6958, -17.925)
  point P32 (-35.6958, -17.925)
  point P33 (-33.9827, -8.9864)
  point P34 (-37.6254, -12.3686)
  point P35 (-4.2815, -8.4793)
  point P36 (-46.4437, 13.615)
  point P37 (-46.4437, 13.615)
  point P38 (-33.4866, 3.3468)
  point P39 (-33.4866, 3.3468)
  point P40 (-36.9741, -24.5955)
  point P41 (-55.791, -24.6391)
  point P42 (-6.1165, -23.9685)
  point P43 (-6.8618, -14.7792)
  point P44 (-6.8618, -14.7792)
  point P45 (-18.7565, -4.9003)
  point P46 (2.4058, -23.9267)
  point P47 (-5.6674, 4.5319)
  point P48 (-5.6674, 4.5319)
  point P49 (-18.7565, -4.9003)
  point P50 (7.7741, -7.0906)
  point P51 (7.7741, -7.0906)
  point P52 (5.9578, -22.7749)
  point P53 (5.9578, -22.7749)
  point P54 (20.3042, -17.925)
  point P55 (20.3042, -17.925)
  point P56 (22.0173, -8.9864)
  point P57 (18.3746, -12.3686)
  point P58 (51.7185, -8.4793)
  point P59 (9.5563, 13.615)
  point P60 (9.5563, 13.615)
  point P61 (22.5134, 3.3468)
  point P62 (22.5134, 3.3468)
  point P63 (19.0259, -24.5955)
  point P64 (0.209, -24.6391)
  point P65 (49.8835, -23.9685)
  point P66 (49.1382, -14.7792)
  point P67 (49.1382, -14.7792)
  point P68 (37.2435, -4.9003)
  point P69 (58.4058, -23.9267)
  point P70 (50.3326, 4.5319)
  point P71 (50.3326, 4.5319)
  point P72 (37.2435, -4.9003)
  point P73 (63.7741, -7.0906)
  point P74 (63.7741, -7.0906)
  point P75 (61.9578, -22.7749)
  point P76 (61.9578, -22.7749)
  point P77 (76.3042, -17.925)
  point P78 (76.3042, -17.925)
  point P79 (78.0173, -8.9864)
  point P80 (74.3746, -12.3686)
  point P81 (107.7185, -8.4793)
  point P82 (65.5563, 13.615)
  point P83 (65.5563, 13.615)
  point P84 (78.5134, 3.3468)
  point P85 (78.5134, 3.3468)
  point P86 (75.0259, -24.5955)
  point P87 (56.209, -24.6391)
  point P88 (73.2385, 11.7133)
  point P89 (17.2385, 11.7133)
  point P90 (-38.7615, 11.7133)
  point P91 (-94.7615, 11.7133)
  point P92 (105.8835, -23.9685)
  point P93 (105.1382, -14.7792)
  point P94 (105.1382, -14.7792)
  point P95 (93.2435, -4.9003)
  point P96 (114.4058, -23.9267)
  point P97 (106.3326, 4.5319)
  point P98 (106.3326, 4.5319)
  point P99 (93.2435, -4.9003)
  point P100 (119.7741, -7.0906)
  point P101 (119.7741, -7.0906)
  point P102 (117.9578, -22.7749)
  point P103 (117.9578, -22.7749)
  point P104 (132.3042, -17.925)
  point P105 (132.3042, -17.925)
  point P106 (134.0173, -8.9864)
  point P107 (130.3746, -12.3686)
  point P108 (163.7185, -8.4793)
  point P109 (121.5563, 13.615)
  point P110 (121.5563, 13.615)
  point P111 (134.5134, 3.3468)
  point P112 (134.5134, 3.3468)
  point P113 (131.0259, -24.5955)
  point P114 (112.209, -24.6391)
  point P115 (129.2385, 11.7133)
  point P116 (-97.8907, -19)
  point P117 (-126.53, -19)
  point P118 (-102.4129, -19)
  point P119 (-99.9271, -19)
  point P120 (-41.8907, -19)
  point P121 (-70.53, -19)
  point P122 (-46.4129, -19)
  point P123 (-43.9271, -19)
  point P124 (14.1093, -19)
  point P125 (70.1093, -19)
  point P126 (41.47, -19)
  point P127 (65.5871, -19)
  point P128 (68.0729, -19)
  point P129 (126.1093, -19)
  point P130 (-46.02, -19.4178)
  point P131 (65.98, -19.4178)
  point P132 (-123.9286, -19)
  point P133 (-114.443, -19)
  point P134 (-11.9286, -19)
  point P135 (-2.443, -19)
  point P136 (44.0714, -19)
  point P137 (53.557, -19)
  point P138 (109.557, -19)
  point P139 (100.0714, -19)
  point P140 (97.47, -19)
  point P141 (121.98, -19.4178)
  point P142 (9.5871, -19)
  point P143 (-14.53, -19)
  point P144 (12.0729, -19)
  point P145 (-102.02, -19.4178)
  point P146 (124.0729, -19)
  point P147 (121.5871, -19)
  point P148 (-67.9286, -19)
  point P149 (-58.443, -19)
  dimension "d0" = 280.8
  dimension "d1" = 50
  dimension "d2" = 55.2
  dimension "d4" = 2
  dimension "d5" = 60
  dimension "d6" = 2
  dimension "d7" = 60
  dimension "d8" = 2
  dimension "d9" = 60
  dimension "d12" = 2
  dimension "d14" = 2
  dimension "d15" = 2
  dimension "d16" = 2
  dimension "d17" = 2
  dimension "d18" = 2
  dimension "d21" = 56
  dimension "d51" = 4
  dimension "d52" = 6
  dimension "d53" = 6
  constraints: 1012 end point, 86 point on line, 50 coincident, 18 parallel, 7 horizontal, 5 midpoint, 2 perpendicular, 1 collinear, 1114 other
  measures "d0" distance of L1.end L2.end
  measures "d1" distance of L0.end L1.end
  measures "d2" distance of L8.end L9.end
  measures "d4" distance between parallel lines of L20 L26
  measures "d5" angle of L20 L31
  measures "d6" distance between parallel lines of L38 L31
  measures "d7" angle of L27 L44
  measures "d8" distance between parallel lines of L50 L44
  measures "d9" angle of L40 L51
  measures "d12" distance between parallel lines of L62 L51
  measures "d14" distance between parallel lines of L67 L72
  measures "d15" distance between parallel lines of L80 L86
  measures "d16" distance between parallel lines of L92 L98
  measures "d17" distance between parallel lines of L99 L110
  measures "d18" distance between parallel lines of L112 L119
  measures "d21" distance of L64.end L147.start
  measures "d51" distance between parallel lines of L11 L8
  measures "d52" distance between parallel lines of L0 L12
extrude "Выдавливание1" add sketch "Эскиз1" along normal blind 4 contours L0 L1 L2 L3 | L57 L62 L61 L14 L56 L51 L11 | L61 L135 L14 | L132 L99 L91 L100 L101 L11 L106 L105 L110 L131 | L41 L42 L43 L44 L39 L40 | L76 L56 L14 | L56 L75 L82 L14 | L136 L82 L75 | L92 L87 L88 L12 L128 L91 | L68 L63 L14 L74 L73 L72 L71 L70 L69 L65 L66 L67 | L82 L75 L14 | L82 L136 L14 L75 | L82 L81 L86 L139 L14 L136 | L28 L29 L30 L31 L32 L27 | L80 L75 L14 L140 | L116 L111 L112 L113 L13 L120 L119 L118 L117 L122 L145 L146 L115 | L15 L13 L21 L125 L12 L126 | L65 L142 L14 | L74 L69 L14 | L232 L235 L147 | L235 L150 L174 L158 L229 L232 L149 L231 L177 L230 L228 L148 | L194 L155 L154 L153 L166 L165 L157 L164 L163 L169 L151 L152 L156 | L232 L149 L148 | L168 L179 L181 L201 L200 L170 | L229 L159 L232 | L210 L213 L195 L184 L172 L173 | L160 L192 L232 L159 | L182 L194 L183 L237 L234 L236 | L205 L220 L234 L215 L209 L207 | L232 L188 L190 L191 L162 L161 | L209 L227 L233 L226 L214 L225 L223 L222 L224 | L197 L233 L198 L199 L186 L232 L187 | L232 L190 L192 | L192 L190 L188 L232 | L232 L189 L187 | L187 L192 L190 L232 | L192 L188 L190 | L232 L186 L193 | L323 L326 L238 | L326 L241 L265 L249 L320 L323 L240 L322 L268 L321 L319 L239 | L285 L246 L245 L244 L257 L256 L248 L255 L254 L260 L242 L243 L247 | L323 L240 L239 | L259 L270 L272 L292 L291 L261 | L301 L304 L286 L275 L263 L264 | L251 L283 L323 L250 | L273 L285 L274 L328 L325 L327 | L296 L311 L325 L306 L300 L298 | L323 L279 L281 L282 L253 L252 | L300 L318 L324 L317 L305 L316 L314 L313 L315 | L288 L324 L289 L290 L277 L323 L278 | L323 L281 L283 | L283 L281 L279 L323 | L323 L280 L278 | L278 L283 L281 L323 | L283 L279 L281 | L323 L277 L284 | L414 L417 L329 | L417 L332 L356 L340 L411 L414 L331 L413 L359 L412 L410 L330 | L376 L337 L336 L335 L348 L347 L339 L346 L345 L351 L333 L334 L338 | L414 L331 L330 | L350 L361 L363 L383 L382 L352 | L392 L395 L377 L366 L354 L355 | L342 L374 L414 L341 | L364 L376 L365 L419 L416 L418 | L387 L402 L416 L397 L391 L389 | L414 L370 L372 L373 L344 L343 | L391 L409 L415 L408 L396 L407 L405 L404 L406 | L379 L415 L380 L381 L368 L414 L369 | L414 L372 L374 | L374 L372 L370 L414 | L414 L371 L369 | L369 L374 L372 L414 | L374 L370 L372 | L414 L368 L375 | L505 L508 L420 | L508 L423 L447 L431 L502 L505 L422 L504 L450 L503 L501 L421 | L467 L428 L427 L426 L439 L438 L430 L437 L436 L442 L424 L425 L429 | L505 L422 L421 | L441 L452 L454 L474 L473 L443 | L483 L486 L468 L457 L445 L446 | L433 L465 L505 L432 | L455 L467 L456 L510 L507 L509 | L478 L493 L507 L488 L482 L480 | L505 L461 L463 L464 L435 L434 | L482 L500 L506 L499 L487 L498 L496 L495 L497 | L470 L506 L471 L472 L459 L505 L460 | L505 L463 L465 | L465 L463 L461 L505 | L505 L462 L460 | L460 L465 L463 L505 | L465 L461 L463 | L505 L459 L466
sketch "Эскиз2" plane through (-140.4, -25, 0) normal (0, -1, 0) x (1, 0, 0)
  line L0 (0, 0) -> (0, 4) projected
  line L1 (6, 4) -> (14.3812, 4) projected
  line L2 (13.1898, 0) -> (6, 0) projected
  line L3 (22, 4) -> (6, 4)
  line L4 (6, 4) -> (6, 0)
  line L5 (6, 0) -> (22, 0)
  line L6 (22, 0) -> (22, 4)
  line L7 (48, 4) -> (32, 4)
  line L8 (32, 4) -> (32, 0)
  line L9 (32, 0) -> (48, 0)
  line L10 (48, 0) -> (48, 4)
  line L11 (74, 4) -> (58, 4)
  line L12 (58, 4) -> (58, 0)
  line L13 (58, 0) -> (74, 0)
  line L14 (74, 0) -> (74, 4)
  line L15 (100, 4) -> (84, 4)
  line L16 (84, 4) -> (84, 0)
  line L17 (84, 0) -> (100, 0)
  line L18 (100, 0) -> (100, 4)
  line L19 (126, 4) -> (110, 4)
  line L20 (110, 4) -> (110, 0)
  line L21 (110, 0) -> (126, 0)
  line L22 (126, 0) -> (126, 4)
  line L23 (152, 4) -> (136, 4)
  line L24 (136, 4) -> (136, 0)
  line L25 (136, 0) -> (152, 0)
  line L26 (152, 0) -> (152, 4)
  line L27 (178, 4) -> (162, 4)
  line L28 (162, 4) -> (162, 0)
  line L29 (162, 0) -> (178, 0)
  line L30 (178, 0) -> (178, 4)
  line L31 (204, 4) -> (188, 4)
  line L32 (188, 4) -> (188, 0)
  line L33 (188, 0) -> (204, 0)
  line L34 (204, 0) -> (204, 4)
  line L35 (230, 4) -> (214, 4)
  line L36 (214, 4) -> (214, 0)
  line L37 (214, 0) -> (230, 0)
  line L38 (230, 0) -> (230, 4)
  line L39 (256, 4) -> (240, 4)
  line L40 (240, 4) -> (240, 0)
  line L41 (240, 0) -> (256, 0)
  line L42 (256, 0) -> (256, 4)
  line L43 (280.8, 4) -> (0, 4) projected
  line L44 (262, 0) -> (274.8, 0)
  line L45 (274.8, 0) -> (274.8, 4)
  line L46 (274.8, 4) -> (262, 4)
  line L47 (262, 4) -> (262, 0)
  line L48 (280.8, 0) -> (280.8, 4) projected
  point P0 (16.4176, 4)
  point P1 (33.6265, 4)
  point P2 (256, 2)
  point P3 (14.4176, 4)
  point P4 (31.6265, 4)
  point P5 (31, 4)
  dimension "d40" = 6
  dimension "d41" = 16
  dimension "d44" = 26
  dimension "d49" = 6
  dimension "d50" = 6
  constraints: 88 end point, 4 parallel, 3 horizontal, 2 perpendicular, 2 point on line, 1 midpoint, 74 other
  measures "d40" distance between parallel lines of L0 L4
  measures "d41" distance of L4.end L5.end
  measures "d44" distance of L3.start L7.start
  measures "d49" distance from line of point (256, 2) L47
  measures "d50" distance between parallel lines of L48 L45
extrude "Выдавливание2" add sketch "Эскиз2" along normal blind 4
mirror "Зеркальное отражение1" about plane through (0, 0, 0) normal (0, 1, 0) of "Выдавливание2"
sketch "Эскиз3" plane through (0, 0, 0) normal (0, 0, -1) x (-1, 0, 0)
  line L0 (-63.6, -25) -> (-73.6, -25) projected
  line L1 (-66.95, -25) -> (-70.25, -25)
  line L2 (-70.25, -25) -> (-70.25, -20)
  line L3 (-70.25, -20) -> (-66.95, -20)
  line L4 (-66.95, -20) -> (-66.95, -25)
  line L5 (-65.9, -23.6) -> (-71.3, -23.6)
  line L6 (-71.3, -23.6) -> (-71.3, -21.3)
  line L7 (-71.3, -21.3) -> (-65.9, -21.3)
  line L8 (-65.9, -21.3) -> (-65.9, -23.6)
  line L9 (66.4, -25) -> (56.4, -25) projected
  line L10 (59.75, -25) -> (63.05, -25)
  line L11 (63.05, -25) -> (63.05, -20)
  line L12 (63.05, -20) -> (59.75, -20)
  line L13 (59.75, -20) -> (59.75, -25)
  line L14 (64.1, -23.6) -> (58.7, -23.6)
  line L15 (58.7, -23.6) -> (58.7, -21.3)
  line L16 (58.7, -21.3) -> (64.1, -21.3)
  line L17 (64.1, -21.3) -> (64.1, -23.6)
  line L18 (-68.6, -25) -> (-68.6, -20) construction
  line L19 (61.4, -25) -> (61.4, -20) construction
  line L20 (-140.4, -25) -> (-140.4, 25) projected
  line L21 (-140.4, 0) -> (140.4, 0) construction
  line L22 (140.4, 25) -> (140.4, -25) construction
  line L23 (-63.6, 25) -> (-73.6, 25)
  line L24 (-66.95, 25) -> (-70.25, 25)
  line L25 (-70.25, 25) -> (-70.25, 20)
  line L26 (-70.25, 20) -> (-66.95, 20)
  line L27 (-66.95, 20) -> (-66.95, 25)
  line L28 (-65.9, 23.6) -> (-71.3, 23.6)
  line L29 (-71.3, 23.6) -> (-71.3, 21.3)
  line L30 (-71.3, 21.3) -> (-65.9, 21.3)
  line L31 (-65.9, 21.3) -> (-65.9, 23.6)
  line L32 (66.4, 25) -> (56.4, 25)
  line L33 (59.75, 25) -> (63.05, 25)
  line L34 (63.05, 25) -> (63.05, 20)
  line L35 (63.05, 20) -> (59.75, 20)
  line L36 (59.75, 20) -> (59.75, 25)
  line L37 (64.1, 23.6) -> (58.7, 23.6)
  line L38 (58.7, 23.6) -> (58.7, 21.3)
  line L39 (58.7, 21.3) -> (64.1, 21.3)
  line L40 (64.1, 21.3) -> (64.1, 23.6)
  line L41 (-68.6, 25) -> (-68.6, 20) construction
  line L42 (61.4, 25) -> (61.4, 20) construction
  line L43 (140.4, -25) -> (140.4, 25) construction
  point P0 (0, 0)
  point P1 (-68.6, -23.6)
  point P2 (61.4, -23.6)
  point P3 (-68.6, 23.6)
  point P4 (61.4, 23.6)
  point P5 (-70.25, 21.3)
  point P6 (-66.95, 21.3)
  point P7 (-66.95, 23.6)
  point P8 (-70.25, 23.6)
  point P9 (-70.25, -23.6)
  point P10 (-66.95, -23.6)
  point P11 (-66.95, -21.3)
  point P12 (-70.25, -21.3)
  point P13 (63.05, 23.6)
  point P14 (59.75, 23.6)
  point P15 (59.75, 21.3)
  point P16 (63.05, 21.3)
  point P17 (59.75, -23.6)
  point P18 (63.05, -23.6)
  point P19 (63.05, -21.3)
  point P20 (59.75, -21.3)
  dimension "d54" = 3.3
  dimension "d55" = 5
  dimension "d56" = 5.4
  dimension "d57" = 2.3
  dimension "d58" = 1.4
  dimension "d59" = 3.3
  dimension "d60" = 5
  dimension "d61" = 5.4
  dimension "d62" = 2.3
  dimension "d63" = 1.4
  constraints: 80 end point, 28 symmetric about line, 10 midpoint, 8 parallel, 8 point on line, 4 horizontal, 4 perpendicular
  measures "d54" distance of L2.end L3.end
  measures "d55" distance of L1.end L2.end
  measures "d56" distance of L6.end L7.end
  measures "d57" distance of L5.end L6.end
  measures "d58" distance between parallel lines of L0 L5
  measures "d59" distance of L11.end L12.end
  measures "d60" distance of L12.end L10.start
  measures "d61" distance of L15.end L16.end
  measures "d62" distance of L14.end L15.end
  measures "d63" distance between parallel lines of L9 L14
extrude "Выдавливание3" cut sketch "Эскиз3" against normal blind 4
